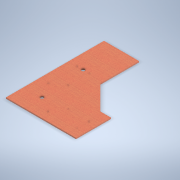
# Autodesk Inventor part: Tapa01
Saved by Autodesk Inventor 2020.3 (Build 243373000, 373)
## iProperties
Created: 2020-10-27
Part Number: Tapa01
Material: Madera (roble)
Document SubType Name: Modeling
Designer: codig
Density: 0.76 g/cm^3
Appearance: Roble blanco - Natural brillo medio
Author: codig
Autodesk Inventor part; units mm, degrees
ref_plane "YZ Plane" through (0, 0, 0) normal (1, 0, 0) x (0, 1, 0)
ref_plane "XZ Plane" through (0, 0, 0) normal (0, 1, 0) x (-1, 0, 0)
ref_plane "XY Plane" through (0, 0, 0) normal (0, 0, 1) x (1, 0, 0)
sketch "Boceto1" plane through (0, 0, 0) normal (0, 1, 0) x (-1, 0, 0)
  line L0 (100, -100) -> (1100, -100)
  line L1 (1100, -100) -> (1100, -1500)
  line L2 (1100, -1500) -> (600, -1500)
  line L3 (100, -600) -> (100, -100)
  line L4 (600, -1500) -> (600, -950)
  line L5 (100, -600) -> (250, -600)
  line L6 (100, -600) -> (250, -600) construction
  line L7 (250, -600) -> (600, -950)
  point P0 (0, 0)
  constraints: 16 end point, 3 horizontal, 2 parallel, 1 collinear, 1 perpendicular
extrude "Extrusión1" add sketch "Boceto1" along normal blind 18
sketch "Boceto2" plane through (0, 0, 0) normal (0, -1, 0) x (1, 0, 0)
  line L0 (-1100, -1500) -> (-1100, -100) projected
  circle A0 centre (-1073, -1132) radius 4
  circle A1 centre (-1073, -800) radius 4
  circle A2 centre (-1073, -468) radius 4
  line L1 (-600, -950) -> (-600, -1500) projected
  circle A3 centre (-734, -1473) radius 4
  circle A4 centre (-850, -1473) radius 4
  circle A5 centre (-966, -1473) radius 4
  line L2 (-100, -100) -> (-100, -600) projected
  circle A6 centre (-359, -127) radius 4
  circle A7 centre (-600, -127) radius 4
  circle A8 centre (-841, -127) radius 4
  point P0 (0, 0)
  constraints: 9 centre point
hole "Agujero1" at (-359, 0, -127) at (-600, 0, -127) at (-841, 0, -127) at (-1073, 0, -468) at (-1073, 0, -800) at (-1073, 0, -1132) at (-734, 0, -1473) at (-850, 0, -1473) at (-966, 0, -1473) direction (0, 1, 0) diameter 8 depth 10
sketch "Boceto3" plane through (0, 0, 0) normal (0, -1, 0) x (1, 0, 0)
  line L0 (-100, -100) -> (-100, -600) projected
  circle A0 centre (-228, -365) radius 4
  circle A1 centre (-338, -365) radius 4
  circle A2 centre (-448, -365) radius 4
  point P0 (0, 0)
  constraints: 3 centre point
hole "Agujero2" at (-448, 0, -365) at (-338, 0, -365) at (-228, 0, -365) direction (0, 1, 0) diameter 8 depth 10
sketch "Boceto4" plane through (0, 0, 0) normal (0, -1, 0) x (1, 0, 0)
  circle A0 centre (-850, -1473) radius 4 projected
  line L0 (-600, -950) -> (-600, -1500) projected
  circle A1 centre (-966, -1473) radius 4 projected
  circle A2 centre (-734, -1055) radius 4
  circle A3 centre (-850, -1055) radius 4
  circle A4 centre (-966, -1055) radius 4
  point P0 (0, 0)
  constraints: 3 centre point
hole "Agujero3" at (-734, 0, -1055) at (-850, 0, -1055) at (-966, 0, -1055) direction (0, 1, 0) diameter 8 depth 10
sketch "Boceto8" plane through (0, 18, 0) normal (0, 1, 0) x (1, 0, 0)
  line L0 (-183.5, 200) -> (-183.5, 420)
  line L1 (-1100, 100) -> (-100, 100) projected
  line L2 (-183.5, 420) -> (-483.5, 420)
  line L3 (-1000, 1016.5) -> (-780, 1016.5)
  line L4 (-1000, 1016.5) -> (-780, 1016.5) construction
  line L5 (-780, 1016.5) -> (-780, 716.5)
  line L6 (-780, 716.5) -> (-483.5, 420)
  line L7 (-1000, 1016.5) -> (-1000, 550)
  line L8 (-183.5, 200) -> (-650, 200)
  line L9 (-650, 200) -> (-1000, 550)
  line L10 (-1000, 1016.5) -> (-964.644, 1016.5) construction
  circle A0 centre (-974.9995, 991.4995) radius 4
  circle A1 centre (-805.0005, 991.4995) radius 4
  circle A2 centre (-974.9995, 575.0005) radius 4
  circle A3 centre (-805.0005, 691.4995) radius 4
  circle A4 centre (-508.5005, 394.9995) radius 4
  circle A5 centre (-624.9995, 225.0005) radius 4
  circle A6 centre (-208.5005, 225.0005) radius 4
  circle A7 centre (-208.5005, 394.9995) radius 4
  circle A8 centre (-208.5005, 394.9995) radius 12.5
  circle A9 centre (-208.5005, 225.0005) radius 12.5
  circle A10 centre (-508.5005, 394.9995) radius 12.5
  circle A11 centre (-624.9995, 225.0005) radius 12.5
  circle A12 centre (-805.0005, 691.4995) radius 12.5
  circle A13 centre (-974.9995, 575.0005) radius 12.5
  circle A14 centre (-974.9995, 991.4995) radius 12.5
  circle A15 centre (-805.0005, 991.4995) radius 12.5
  circle A16 centre (-890, 991.4995) radius 25
  circle A17 centre (-842.6777, 357.3223) radius 25
  point P0 (0, 0)
  constraints: 20 end point, 18 centre point, 8 coincident, 4 horizontal, 3 perpendicular, 1 collinear
hole "Agujero7" at (-805.0005, 18, -991.4995) at (-974.9995, 18, -991.4995) at (-805.0005, 18, -691.4995) at (-974.9995, 18, -575.0005) at (-508.5005, 18, -394.9995) at (-624.9995, 18, -225.0005) at (-208.5005, 18, -225.0005) at (-208.5005, 18, -394.9995) direction (0, -1, 0) diameter 8 end through all counterbore diameter 25 counterbore depth 2
hole "Agujero8" at (-842.6777, 18, -357.3223) at (-890, 18, -991.4995) direction (0, -1, 0) diameter 50 end through all
